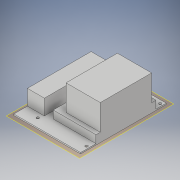
# Autodesk Inventor part: jetson
Saved by Autodesk Inventor 2019 (Build 230136000, 136)
## iProperties
Created: 2021-05-27
Part Number: jetson
Material: Generisch
Document SubType Name: Modeling
Designer: Lukas
Density: 1 g/cm^3
Appearance: Vorgabe
Author: Lukas
Autodesk Inventor part; units mm, degrees
ref_plane "YZ Plane" through (0, 0, 0) normal (1, 0, 0) x (0, 1, 0)
ref_plane "XY Plane" through (0, 0, 0) normal (0, 0, 1) x (1, 0, 0)
sketch "Skizze1" plane through (0, 0, 0) normal (0, 1, 0) x (-1, 0, 0)
  line L0 (0, 0) -> (-78, 0)
  line L1 (-78, 0) -> (-78, -100)
  line L2 (-78, -100) -> (0, -100)
  line L3 (0, -100) -> (0, 0)
  dimension "d0" = 78
  dimension "d1" = 100
  constraints: 8 end point, 2 parallel, 1 coincident, 1 horizontal, 1 perpendicular
  measures "d0" distance of L2.end L1.end
  measures "d1" distance of L1.end L0.end
extrude "Extrusion1" add sketch "Skizze1" along normal blind 1.5
sketch "Skizze2" plane through (0, 1.5, 0) normal (0, 1, 0) x (1, 0, 0)
  line L0 (78, 100) -> (0, 100) projected
  line L1 (78, 0) -> (78, 100) projected
  line L2 (0, 0) -> (78, 0) projected
  line L3 (0, 100) -> (0, 0) projected
  point P0 (75, 96)
  point P1 (75, 10)
  point P2 (18, 10)
  point P3 (18, 96)
  dimension "d4" = 4
  dimension "d5" = 3
  dimension "d6" = 10
  dimension "d7" = 3
  dimension "d8" = 18
  dimension "d9" = 10
  dimension "d10" = 4
  dimension "d11" = 18
  measures "d4" distance from line of L0 point (75, 96)
  measures "d5" distance from line of L1 point (75, 96)
  measures "d6" distance from line of L2 point (75, 10)
  measures "d7" distance from line of L1 point (75, 10)
  measures "d8" distance from line of L3 point (18, 10)
  measures "d9" distance from line of L2 point (18, 10)
  measures "d10" distance from line of L0 point (18, 96)
  measures "d11" distance from line of L3 point (18, 96)
hole "Bohrung1" at (75, 1.5, -96) at (75, 1.5, -10) at (18, 1.5, -10) at (18, 1.5, -96) direction (0, -1, 0) diameter 3 end through all
sketch "Skizze3" plane through (0, 1.5, 0) normal (0, 1, 0) x (1, 0, 0)
  line L0 (0, 100) -> (0, 0) projected
  line L1 (0, 15.8637) -> (19.8459, 15.8637)
  line L2 (19.8459, 15.8637) -> (19.8459, 90.2858)
  line L3 (19.8459, 90.2858) -> (0, 90.2858)
  line L4 (0, 90.2858) -> (0, 15.8637)
  dimension "d19" = 15.8637
  dimension "d20" = 74.4222
  dimension "d21" = 19.8459
  constraints: 8 end point, 2 parallel, 1 horizontal, 1 perpendicular, 1 point on line
  measures "d19" distance of L0.end L1.start
  measures "d20" distance of L1.end L2.end
  measures "d21" distance of L2.end L3.end
extrude "Extrusion2" add sketch "Skizze3" along normal blind 18
sketch "Skizze4" plane through (0, 1.5, 0) normal (0, 1, 0) x (1, 0, 0)
  line L0 (78, 0) -> (78, 100) projected
  line L1 (78, 18) -> (28, 18)
  line L2 (28, 18) -> (28, 88)
  line L3 (28, 88) -> (78, 88)
  line L4 (78, 88) -> (78, 18)
  line L5 (0, 0) -> (78, 0) projected
  dimension "d24" = 18
  dimension "d25" = 50
  dimension "d26" = 70
  constraints: 8 end point, 2 parallel, 1 horizontal, 1 perpendicular, 1 point on line
  measures "d24" distance between parallel lines of L5 L1
  measures "d25" distance of L2.end L3.end
  measures "d26" distance of L1.end L2.end
extrude "Extrusion3" add sketch "Skizze4" along normal blind 9
sketch "Skizze5" plane through (0, 10.5, 0) normal (0, 1, 0) x (1, 0, 0)
  line L0 (38, 23.0032) -> (78, 23.0032)
  line L1 (78, 23.0032) -> (78, 83.0032)
  line L2 (78, 83.0032) -> (38, 83.0032)
  line L3 (38, 83.0032) -> (38, 23.0032)
  line L4 (78, 18) -> (78, 88) projected
  line L5 (28, 18) -> (78, 18) projected
  point P0 (0, 0)
  dimension "d29" = 40
  dimension "d30" = 60
  dimension "d31" = 5.0032
  constraints: 8 end point, 2 parallel, 1 horizontal, 1 perpendicular, 1 point on line
  measures "d29" distance of L2.end L1.end
  measures "d30" distance of L1.end L0.end
  measures "d31" distance between parallel lines of L5 L0
extrude "Extrusion4" add sketch "Skizze5" along normal blind 30
